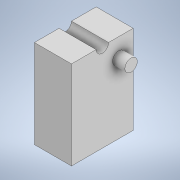
# Autodesk Inventor part: Support_1A
Saved by Autodesk Inventor 2021 (Build 250183000, 183)
## iProperties
Created: 2021-04-14
Part Number: Support_1A
Material: Generic
Document SubType Name: Modeling
Designer: Jawal
Density: 1 g/cm^3
Appearance: Default
Author: Jawal
Autodesk Inventor part; units mm, degrees
ref_plane "YZ Plane" through (0, 0, 0) normal (1, 0, 0) x (0, 1, 0)
ref_plane "XZ Plane" through (0, 0, 0) normal (0, 1, 0) x (-1, 0, 0)
ref_plane "XY Plane" through (0, 0, 0) normal (0, 0, 1) x (1, 0, 0)
sketch "Sketch1" plane through (0, 0, 0) normal (1, 0, 0) x (0, 1, 0)
  line L0 (10.7385, 7.5) -> (-10.7385, 7.5)
  line L1 (-10.7385, 7.5) -> (-10.7385, -7.5)
  line L2 (-10.7385, -7.5) -> (10.7385, -7.5)
  line L3 (10.7385, -7.5) -> (10.7385, 7.5)
  point P0 (0, 0)
  dimension "d0" = 21.477
  dimension "d1" = 15
  dimension "d2" = 10.7385
  dimension "d3" = 7.5
  constraints: 8 end point, 2 parallel, 1 horizontal, 1 perpendicular
  measures "d0" distance of L1.end L2.end
  measures "d1" distance of L2.end L0.start
  measures "d2" distance from line of L3 point (0, 0)
  measures "d3" distance from line of L0 point (0, 0)
extrude "Extrusion1" add sketch "Sketch1" along normal blind 9
sketch "Sketch2" plane through (9, 0, 0) normal (1, 0, 0) x (0, 0, -1)
  line L0 (7.5, 10.7385) -> (-7.5, 10.7385) projected
  arc A0 (-1.5, 10.7385) -> (1.5, 10.7385) centre (0, 10.7385) ccw
  point P0 (0, 0)
  dimension "d8" = 3
  constraints: 2 point on circle, 2 point on line, 1 centre point, 1 midpoint
  measures "d8" diameter of A0
extrude "Extrusion2" cut sketch "Sketch2" against normal through all
sketch "Sketch3" plane through (9, 0, 0) normal (1, 0, 0) x (0, 0, -1)
  circle A0 centre (3.983, 6.2605) radius 1.5
  arc A1 (-1.5, 10.7385) -> (1.5, 10.7385) centre (0, 10.7385) ccw projected
  line L0 (7.5, 10.7385) -> (1.5, 10.7385) projected
  point P0 (0, 0)
  dimension "d12" = 3
  dimension "d13" = 3.983
  dimension "d14" = 4.478
  constraints: 1 centre point
  measures "d12" diameter of A0
  measures "d13" horizontal distance of A1.centre A0.centre
  measures "d14" distance from line of L0 A0.centre
extrude "Extrusion3" add sketch "Sketch3" along normal blind 3
equation "\"d2\" = 0.5 * d0"
body "Solid1"
